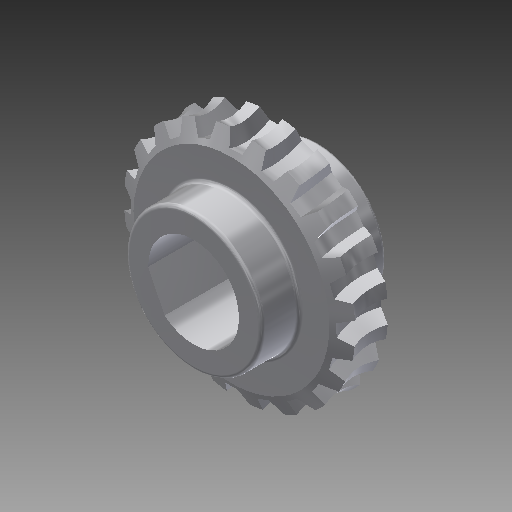
# Autodesk Inventor part: 401-03
Saved by Autodesk Inventor 2019 (Build 230136000, 136)
## iProperties
Created: 2007-11-19
Part Number: 401-03
Material: Acetal Resin, White
Document SubType Name: Modeling
Designer: Autodesk Inc.
Density: 1.425 g/cm^3
Mass: 6.64879 g
Surface Area: 30.2026 cm^2
Volume: 4.66582 cm^3
Description: WORM GEAR - 20 TOOTH
Appearance: Smooth - White
CustomPartVersion: 1
Company: Autodesk Inc.
Component Category: Lower Component
d69: 20.000 mm
d74: 0.000 mm
d87: 0.000 mm
d88: 0.000 mm
d89: 0.000 mm
d95: 20.000 mm
d96: 0.000 mm
d97: 0.000 mm
Author: Inventor
Autodesk Inventor part; units mm, degrees
ref_plane "Tooth Plane" through (0, -10, 0) normal (-0.0995037, 0, 0.9950372) x (0, 1, 0)
sketch "Base Body Sketch" plane through (0, 0, 0) normal (1, 0, 0) x (0, 1, 0)
  line L0 (0, -10.1438) -> (0, 10.1438) projected
  line L1 (0, 3.25) -> (12.9515, 3.25)
  line L2 (0, 3.25) -> (0, -3.25)
  line L3 (0, -3.25) -> (12.9515, -3.25)
  line L4 (12.9515, 3.25) -> (15.301, 2.1667)
  line L5 (12.9515, -3.25) -> (15.301, -2.1667)
  arc A0 (15.301, 2.1667) -> (15.301, -2.1667) centre (20, 0) ccw
  line L6 (-4.9237, 0) -> (24.154, 0) projected
  circle A1 centre (6.4758, 0) radius 7.2456 construction
  dimension "d30" = 49.508
  dimension "d31" = 5.1745
  dimension "d32" = 6.5
  dimension "d33" = 20
  dimension "d50" = 24.754
  constraints: 10 end point, 6 point on circle, 3 perpendicular, 3 point on line, 2 centre point, 1 collinear
  measures "d30" angle of L5 L4
  measures "d31" radius of A0
  measures "d32" distance of L1.start L2.end
  measures "d33" distance from line of L0 A0.centre
  measures "d50" angle of L4 L1
revolve "Base Body" add sketch "Base Body Sketch" angle 360 about axis through (0, 0, 0) along (0, 0, 1)
sketch "Tooth Sketch" plane through (0, -10, 0) normal (-0.0995037, 0, 0.9950372) x (0, 1, 0)
  line L0 (10, 2.2594) -> (10, -2.2594) projected
  line L1 (-11.4169, 0) -> (-1.4989, 0) projected
  line L2 (-10, 1.6138) -> (-10, -1.6138)
  line L3 (-10, -1.6138) -> (-5.0843, -1.6138)
  line L4 (-5.0843, -1.6138) -> (-2.9157, -0.8246)
  line L5 (-2.9157, -0.8246) -> (-2.9157, 0)
  line L6 (-2.9157, 0.8246) -> (-5.0843, 1.6138)
  line L7 (-5.0843, 1.6138) -> (-10, 1.6138)
  line L8 (-2.9157, 0.8246) -> (-2.9157, 0)
  line L9 (-4, 0) -> (-4, -1.2192) construction
  dimension "d38" = 20
  dimension "d39" = 20
  dimension "d40" = 4.9157
  dimension "d41" = 6
  dimension "d42" = 1.2192
  constraints: 16 end point, 4 perpendicular, 3 equal length, 2 point on line, 1 midpoint, 1 parallel, 1 vertical
  measures "d38" distance between parallel lines of L0 L2
  measures "d39" angle of L6 L7
  measures "d40" distance of L6.end L2.start
  measures "d41" distance between parallel lines of L2 L9
  measures "d42" distance of L9.start L9.end
sketch "Sketch10" plane through (0, 0, 3.25) normal (0, 0, 1) x (1, 0, 0)
  circle A0 centre (0, 0) radius 12.9515 projected
  circle A1 centre (0, 0) radius 13.5
  dimension "d81" = 27
  constraints: 1 centre point, 1 coincident
  measures "d81" diameter of A1
surface extrude "ExtrusionSrf1" sketch "Sketch10" against normal blind 6.5 shown no curves A1
revolve "Tooth" cut sketch "Tooth Sketch" angle 360 about axis through (-1.6058, -20, -0.1606) along (0.9950372, 0, 0.0995037)
pattern_circular "Tooth Pattern" count 20 over 360 about axis through (0, 0, 0) along (0, 0, 1) of "Tooth"
ref_plane "Work Plane15" through (0, 0, 0) normal (0.9876883, 0.1564345, 0) x (0, 0, 1)
ref_plane "Work Plane16" through (0, 0, 0) normal (0, -1, 0) x (0, 0, 1)
sketch "Sketch11" plane through (0, 0, -3.25) normal (0, 0, -1) x (-1, 0, 0)
  arc A0 (5.9991, -0.1059) -> (3.8358, -4.6137) centre (0, 0) ccw projected
  line L0 (3.8358, -4.6137) -> (5.9991, -0.1059) projected
  arc A1 (6.0986, -0.1296) -> (6.0986, -0.1296) centre (0, 0) ccw
  line L1 (6.0986, -0.1296) -> (6.0986, -0.1296)
  dimension "d101" = 0.1
  constraints: 2 end point, 2 point on circle, 1 centre point, 1 other
  measures "d101" radial gap between concentric circles of A0 A1
extrude "Extrusion1" cut sketch "Sketch11" against normal through all contours L0 A0
sketch "Sketch12" plane through (0, 0, -3.25) normal (0, 0, -1) x (-1, 0, 0)
  line L0 (5.9991, -0.1059) -> (3.8358, -4.6137) projected
  arc A0 (5.9991, -0.1059) -> (3.8358, -4.6137) centre (0, 0) ccw projected
  circle A1 centre (0, 0) radius 12.9515 projected
  circle A2 centre (0, 0) radius 9
  point P0 (-5.2093, -11.8577)
  point P1 (-2.7553, -12.655)
  point P2 (6.4569, 11.1066)
  point P3 (7.5068, 10.5542)
  dimension "d103" = 18
  constraints: 1 centre point, 1 coincident, 1 other
  measures "d103" diameter of A2
extrude "Extrusion2" add sketch "Sketch12" along normal blind 5 contours A2
mirror "Mirror1" about plane through (0, 0, 0) normal (0, 0, 1) of "Extrusion2"
fillet "Fillet1" radius 0.5 4 edges at (9, 0, 8.25) (9, 0, 3.25) (9, 0, -3.25) (9, 0, -8.25)
equation "\"d30\" = 2 * da_fi"
equation "\"d31\" = da_aw - 0.5 * da_da"
equation "\"d32\" = da_b"
equation "\"d33\" = da_aw"
equation "\"d50\" = da_fi"
equation "\"d38\" = da_aw"
equation "\"d39\" = da_alfat"
equation "\"d40\" = 0.5 * da_df1"
equation "\"d42\" = 0.3 * da_px"
equation "\"d82\" = da_b"
equation "\"da_aw\" = 20"
equation "\"da_fi\" = 24.7541deg"
equation "\"da_b\" = 6.5"
equation "\"da_df\" = 23.95922"
equation "\"da_da\" = 29.65111"
equation "\"da_beta\" = 5.710593deg"
equation "\"da_alfat\" = 20deg"
equation "\"da_df1\" = 9.83145"
equation "\"da_da1\" = 15.52334"
equation "\"da_d1\" = 12.93611"
equation "\"da_px\" = 4.064"
equation "\"d69\" = da_aw"
equation "\"da_dw\" = 25.87223"
equation "\"da_rightdir\" = 0"
equation "\"d95\" = da_aw"
body "Solid1"
body "Srf1"
